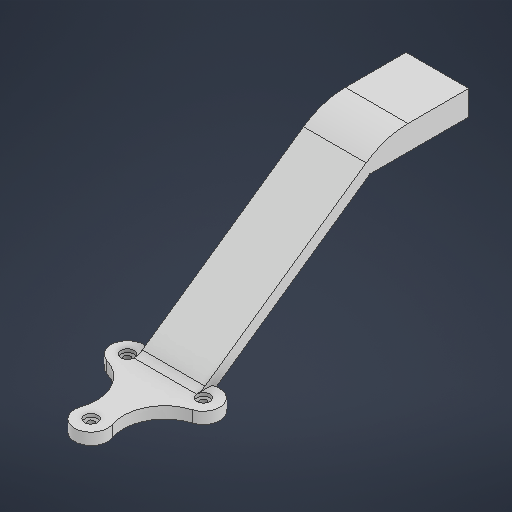
# Autodesk Inventor part: 라이다 고
Saved by Autodesk Inventor 2026.2 (Build 302298000, 298)
## iProperties
Created: 2025-11-27
Part Number: 라이다 고
Material: 일반
Document SubType Name: Modeling
Designer: PC
Density: 1 g/cm^3
Appearance: 기본값
Author: PC
Autodesk Inventor part; units mm, degrees
ref_plane "YZ Plane" through (0, 0, 0) normal (1, 0, 0) x (0, 1, 0)
ref_plane "XZ Plane" through (0, 0, 0) normal (0, 1, 0) x (-1, 0, 0)
ref_plane "XY Plane" through (0, 0, 0) normal (0, 0, 1) x (1, 0, 0)
sketch "스케치1" plane through (0, 0, 0) normal (0, 1, 0) x (-1, 0, 0)
  circle A0 centre (0, 0) radius 2
  line L0 (0, 0) -> (0, -45)
  line L1 (23, -45) -> (-23, -45)
  circle A1 centre (23, -45) radius 2
  circle A2 centre (-23, -45) radius 2
  circle A3 centre (23, -45) radius 10
  circle A4 centre (-23, -45) radius 10
  circle A5 centre (0, 0) radius 10
  arc A6 (9.447, -3.2795) -> (25.8755, -35.4224) centre (33.0643, -11.4782) ccw
  line L2 (0, -115.952) -> (0, 30.992) projected
  arc A7 (-25.8755, -35.4224) -> (-9.447, -3.2795) centre (-33.0643, -11.4782) ccw
  arc A8 (18.8182, -54.0836) -> (-18.8182, -54.0836) centre (0, -94.96) ccw
  point P0 (-9.447, -3.2795)
  point P1 (-25.8755, -35.4224)
  dimension "d6" = 20
  dimension "d7" = 20
  dimension "d0" = 4
  dimension "d1" = 45
  dimension "d2" = 46
  dimension "d3" = 4
  dimension "d4" = 4
  dimension "d5" = 20
  dimension "d8" = 25
  dimension "d9" = 45
  constraints: 8 point on circle, 7 centre point, 6 coincident, 4 end point, 3 symmetric about line, 2 tangent, 1 horizontal, 1 midpoint, 1 vertical, 9 other
  measures "d0" diameter of A0
  measures "d1" distance of L0.end L0.start
  measures "d2" distance of L1.start L1.end
  measures "d3" diameter of A1
  measures "d4" diameter of A2
  measures "d5" diameter of A3
  measures "d8" radius of A6
  measures "d9" radius of A8
extrude "돌출1" add sketch "스케치1" along normal blind 5 contours A0 L2 A5 L0 | A0 L0 A5 L2 | A5 A6 A3 L1 L0 | L0 L1 A4 A7 A5 | L2 A8 A4 L1 | L1 A3 A8 L2 | A4 | A3
sketch "스케치2" plane through (0, 5, 0) normal (0, 1, 0) x (1, 0, 0)
  arc A0 (-9.447, 3.2795) -> (9.447, 3.2795) centre (0, 0) ccw projected
  arc A1 (25.8755, 35.4224) -> (9.447, 3.2795) centre (33.0643, 11.4782) ccw projected
  arc A2 (25.8755, 35.4224) -> (18.8182, 54.0836) centre (23, 45) ccw projected
  arc A3 (-18.8182, 54.0836) -> (18.8182, 54.0836) centre (0, 94.96) ccw projected
  arc A4 (-18.8182, 54.0836) -> (-25.8755, 35.4224) centre (-23, 45) ccw projected
  arc A5 (-9.447, 3.2795) -> (-25.8755, 35.4224) centre (-33.0643, 11.4782) ccw projected
  circle A6 centre (-23, 45) radius 2 projected
  circle A7 centre (23, 45) radius 2 projected
  circle A8 centre (0, 0) radius 2 projected
  circle A9 centre (-23, 45) radius 4
  circle A10 centre (23, 45) radius 4
  circle A11 centre (0, 0) radius 4
  dimension "d12" = 8
  dimension "d13" = 8
  dimension "d14" = 8
  constraints: 3 centre point, 3 coincident
  measures "d12" diameter of A9
  measures "d13" diameter of A10
  measures "d14" diameter of A11
extrude "돌출2" add sketch "스케치2" along normal blind 2 contours A5 A4 A3 A2 A1 A0
sketch "스케치7" plane through (0, 0, 0) normal (1, 0, 0) x (0, 1, 0)
  line L0 (5, -43) -> (5, -47) projected
  line L1 (0, -43) -> (0, -47) projected
  line L2 (7, -41) -> (7, -49) projected
  line L3 (5, -49) -> (5, -41) projected
  line L4 (0, -45) -> (7, -45)
  line L5 (7, -41) -> (7, -49) projected
  line L6 (7, -45) -> (0, -45)
  line L7 (7, -55) -> (7, -35.4224) projected
  line L8 (0, -49.96) -> (0, -54.0836) projected
  line L9 (0, -45) -> (0, -49.96)
  line L10 (0, -49.96) -> (70, -150)
  line L11 (77, -147.7942) -> (8.6259, -50.0779)
  arc A0 (7, -44.9181) -> (8.6259, -50.0779) centre (16, -44.9181) ccw
  line L12 (77, -147.7942) -> (77, -210)
  line L13 (70, -150) -> (70, -210)
  line L14 (77, -210) -> (70, -210)
  line L15 (77, -210) -> (85, -210)
  line L16 (85, -210) -> (85, -173.1814)
  arc A1 (85, -173.1814) -> (77, -147.7942) centre (40.718, -173.1814) ccw
  point P0 (0, 0)
  point P1 (7, -54.0836)
  point P2 (7, -44.9181)
  dimension "d34" = 7
  dimension "d35" = 9
  dimension "d36" = 7
  dimension "d37" = 60
  dimension "d39" = 165
  dimension "d40" = 70
  dimension "d41" = 8
  constraints: 20 end point, 4 point on circle, 4 tangent, 4 vertical, 3 horizontal, 3 midpoint, 2 centre point, 1 parallel, 1 point on line
  measures "d34" distance between parallel lines of L10 L11
  measures "d35" radius of A0
  measures "d36" distance between parallel lines of L12 L13
  measures "d37" distance of L10.end L13.end
  measures "d39" distance between parallel lines of L4 L14
  measures "d40" distance between parallel lines of L9 L13
  measures "d41" distance of L12.end L15.end
extrude "돌출7" add sketch "스케치7" along normal mid plane 38
sketch "스케치8" plane through (19, 85, -210) normal (0, 0, -1) x (-1, 0, 0)
  line L0 (38, -15) -> (0, -15) projected
  line L1 (19, -15) -> (19, -8)
  line L2 (38, -8) -> (0, -8) projected
  line L3 (9, -10) -> (29, -10)
  circle A0 centre (9, -10) radius 2
  circle A1 centre (29, -10) radius 2
  line L4 (38, 0) -> (0, 0) projected
  point P0 (19, -85)
  point P1 (19, -10)
  dimension "d44" = 20
  dimension "d45" = 4
  dimension "d46" = 4
  dimension "d47" = 10
  constraints: 4 end point, 3 midpoint, 2 centre point, 2 coincident, 1 horizontal, 1 point on line
  measures "d44" distance of L3.start L3.end
  measures "d45" diameter of A0
  measures "d46" diameter of A1
  measures "d47" distance from line of L4 point (19, -10)
extrude "돌출8" cut sketch "스케치8" against normal blind 25 contours A0 | A1
